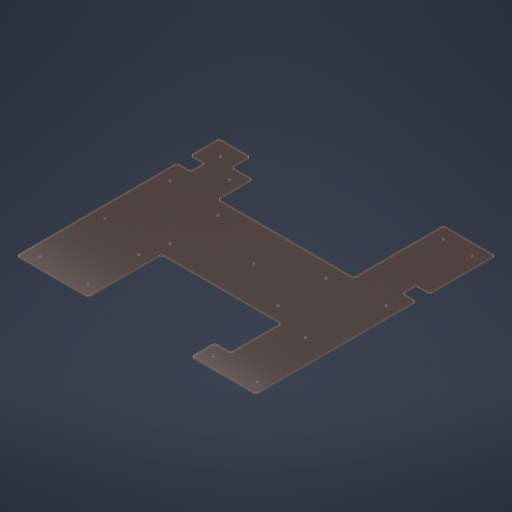
# Autodesk Inventor part: DB1-023
Saved by Autodesk Inventor 2023.4 (Build 274418000, 418)
## iProperties
Created: 2025-03-10
Part Number: DB1-023
Material: Polycarbonate, Smoke
Document SubType Name: Sheet Metal
Designer: brand
Density: 1.2 g/cm^3
Sheet Metal Rule: Default
Appearance: Polycarbonate - Smoked
Author: brand
Autodesk Inventor part; units mm, degrees
ref_plane "YZ Plane" through (0, 0, 0) normal (1, 0, 0) x (0, 1, 0)
ref_plane "XZ Plane" through (0, 0, 0) normal (0, 1, 0) x (-1, 0, 0)
ref_plane "XY Plane" through (0, 0, 0) normal (0, 0, 1) x (1, 0, 0)
sketch "Sketch1" plane through (0, 0, 0) normal (0, 1, 0) x (-1, 0, 0)
  line L0 (329.819, 329.819) -> (-329.819, 329.819)
  line L1 (-329.819, 329.819) -> (-329.819, -329.819)
  line L2 (-329.819, -329.819) -> (329.819, -329.819)
  line L3 (329.819, -329.819) -> (329.819, 329.819)
  line L4 (329.819, 329.819) -> (-329.819, -329.819) construction
  line L5 (-329.819, 329.819) -> (329.819, -329.819) construction
  line L6 (133.35, 329.819) -> (-133.35, 329.819) construction
  line L7 (-133.35, 329.819) -> (-133.35, 126.619)
  line L8 (-133.35, 126.619) -> (133.35, 126.619)
  line L9 (133.35, 126.619) -> (133.35, 329.819)
  line L10 (187.325, -329.819) -> (-187.325, -329.819) construction
  line L11 (-187.325, -329.819) -> (-187.325, -82.169)
  line L12 (-187.325, -82.169) -> (187.325, -82.169)
  line L13 (187.325, -82.169) -> (187.325, -329.819)
  point P0 (0, 0)
  point P1 (0, 329.819)
  point P2 (0, 329.819)
  point P3 (0, -329.819)
  point P4 (0, -329.819)
  point P5 (-133.35, 329.819)
  dimension "d0" = 659.638
  dimension "d1" = 659.638
  dimension "d2" = 266.7
  dimension "d3" = 203.2
  dimension "d4" = 247.65
  dimension "d5" = 374.65
  constraints: 28 end point, 6 midpoint, 6 parallel, 3 horizontal, 3 perpendicular, 2 coincident, 2 point on line
  measures "d0" distance of L0.start L0.end
  measures "d1" distance of L2.end L0.start
  measures "d2" distance of L7.end L8.end
  measures "d3" distance of L8.end L6.start
  measures "d4" distance of L12.end L10.start
  measures "d5" distance of L11.end L12.end
extrude "Extrusion1" add sketch "Sketch1" along normal mid plane 3.175 contours L3 L2 L13 L12 L11 L1 L0 L7 L8 L9
sketch "Sketch2" plane through (0, 1.5875, 0) normal (0, 1, 0) x (1, 0, 0)
  circle A0 centre (-283.3124, 275.8316) radius 34.925 construction
  line L0 (329.819, 329.819) -> (329.819, -329.819) construction
  line L1 (329.819, -329.819) -> (133.35, -329.819) construction
  line L2 (133.35, -329.819) -> (133.35, -126.619) construction
  line L3 (133.35, -126.619) -> (-133.35, -126.619) construction
  line L4 (-133.35, -126.619) -> (-133.35, -329.819) construction
  line L5 (-133.35, -329.819) -> (-329.819, -329.819) construction
  line L6 (-329.819, -329.819) -> (-329.819, 329.819) construction
  line L7 (-329.819, 329.819) -> (-187.325, 329.819) construction
  line L8 (-187.325, 329.819) -> (-187.325, 82.169) construction
  line L9 (-187.325, 82.169) -> (187.325, 82.169) construction
  line L10 (187.325, 82.169) -> (187.325, 329.819) construction
  line L11 (187.325, 329.819) -> (329.819, 329.819) construction
  line L12 (-187.325, 329.819) -> (-329.819, 329.819) construction
  line L13 (-329.819, 329.819) -> (-187.325, 329.819)
  line L14 (-187.325, 329.819) -> (-187.325, 228.219)
  line L15 (-187.325, 228.219) -> (-329.819, 228.219)
  line L16 (-329.819, 228.219) -> (-329.819, 329.819)
  line L17 (329.819, -329.819) -> (133.35, -329.819) construction
  line L18 (133.35, -126.619) -> (152.4, -126.619)
  line L19 (152.4, -126.619) -> (152.4, -329.819)
  line L20 (152.4, -329.819) -> (133.35, -329.819)
  line L21 (133.35, -329.819) -> (133.35, -126.619)
  line L22 (-329.819, 329.819) -> (-329.819, -329.819) construction
  line L23 (-329.819, 149.606) -> (-291.719, 149.606)
  line L24 (-291.719, 149.606) -> (-291.719, 111.506)
  line L25 (-291.719, 111.506) -> (-329.819, 111.506)
  line L26 (-329.819, 111.506) -> (-329.819, 149.606)
  line L27 (329.819, 149.606) -> (291.719, 149.606)
  line L28 (291.719, 149.606) -> (291.719, 111.506)
  line L29 (291.719, 111.506) -> (329.819, 111.506)
  line L30 (329.819, 111.506) -> (329.819, 149.606)
  line L31 (152.4, -126.619) -> (196.85, -126.619)
  line L32 (196.85, -126.619) -> (196.85, -266.319)
  line L33 (196.85, -266.319) -> (152.4, -266.319)
  line L34 (152.4, -266.319) -> (152.4, -126.619)
  line L35 (-187.325, 82.169) -> (-187.325, 329.819) construction
  line L36 (-187.325, 228.219) -> (-244.475, 228.219)
  line L37 (-244.475, 228.219) -> (-244.475, 177.419)
  line L38 (-244.475, 177.419) -> (-187.325, 177.419)
  line L39 (-187.325, 177.419) -> (-187.325, 228.219)
  circle A1 centre (-219.075, 209.169) radius 19.05 construction
  point P0 (0, 0)
  point P1 (-329.819, 130.556)
  point P2 (152.4, -266.319)
  dimension "d9" = 69.85
  dimension "d10" = 46.5066
  dimension "d11" = 53.9874
  dimension "d12" = 101.6
  dimension "d16" = 19.05
  dimension "d17" = 460.375
  dimension "d18" = 38.1
  dimension "d19" = 38.1
  dimension "d20" = 63.5
  dimension "d21" = 63.5
  dimension "d28" = 38.1
  dimension "d29" = 31.75
  dimension "d30" = 120.65
  dimension "d31" = 57.15
  dimension "d32" = 50.8
  constraints: 48 end point, 13 parallel, 6 horizontal, 6 perpendicular, 4 point on line, 2 centre point, 2 horizontal alignment, 1 midpoint
  measures "d9" diameter of A0
  measures "d10" distance from line of L16 A0.centre
  measures "d11" distance from line of L7 A0.centre
  measures "d12" distance of L13.end L14.end
  measures "d16" distance of L2.end L18.end
  measures "d17" distance from line of L5 point (-329.819, 130.556)
  measures "d18" distance of L23.end L24.end
  measures "d19" distance of L24.end L25.end
  measures "d20" distance between parallel lines of L2 L32
  measures "d21" distance between parallel lines of L1 L33
  measures "d28" diameter of A1
  measures "d29" distance from line of L35 A1.centre
  measures "d30" distance from line of L7 A1.centre
  measures "d31" distance of L37.end L38.end
  measures "d32" distance of L36.end L37.end
extrude "Extrusion2" cut sketch "Sketch2" against normal through all
fillet "Fillet1" radius 5.715 24 edges at (-133.35, 0, 126.619) (329.819, 0, 329.819) (329.819, 0, -329.819) (187.325, 0, -329.819) (187.325, 0, -82.169) (-187.325, 0, -82.169) (-329.819, 0, 329.819) (-329.819, 0, -228.219) (152.4, 0, 329.819) (-329.819, 0, -149.606) (-291.719, 0, -149.606) (-291.719, 0, -111.506) (-329.819, 0, -111.506) (291.719, 0, -149.606) (291.719, 0, -111.506) (329.819, 0, -111.506) (329.819, 0, -149.606) (196.85, 0, 126.619) (196.85, 0, 266.319) (152.4, 0, 266.319) (-187.325, 0, -177.419) (-244.475, 0, -177.419) (-244.475, 0, -228.219) (-133.35, 0, 329.819)
sketch "Sketch4" plane through (0, 1.5875, 0) normal (0, 1, 0) x (1, 0, 0)
  arc A0 (324.104, -329.819) -> (329.819, -324.104) centre (324.104, -324.104) ccw construction
  line L0 (324.104, -329.819) -> (158.115, -329.819) construction
  arc A1 (152.4, -324.104) -> (158.115, -329.819) centre (158.115, -324.104) ccw construction
  line L1 (152.4, -324.104) -> (152.4, -272.034) construction
  arc A2 (158.115, -266.319) -> (152.4, -272.034) centre (158.115, -272.034) ccw construction
  line L2 (158.115, -266.319) -> (191.135, -266.319) construction
  arc A3 (191.135, -266.319) -> (196.85, -260.604) centre (191.135, -260.604) ccw construction
  line L3 (196.85, -260.604) -> (196.85, -132.334) construction
  arc A4 (196.85, -132.334) -> (191.135, -126.619) centre (191.135, -132.334) ccw construction
  line L4 (191.135, -126.619) -> (-127.635, -126.619) construction
  arc A5 (-127.635, -126.619) -> (-133.35, -132.334) centre (-127.635, -132.334) ccw construction
  line L5 (-133.35, -132.334) -> (-133.35, -324.104) construction
  arc A6 (-139.065, -329.819) -> (-133.35, -324.104) centre (-139.065, -324.104) ccw construction
  line L6 (-139.065, -329.819) -> (-324.104, -329.819) construction
  arc A7 (-329.819, -324.104) -> (-324.104, -329.819) centre (-324.104, -324.104) ccw construction
  line L7 (-329.819, -324.104) -> (-329.819, 105.791) construction
  arc A8 (-324.104, 111.506) -> (-329.819, 105.791) centre (-324.104, 105.791) ccw construction
  line L8 (-324.104, 111.506) -> (-297.434, 111.506) construction
  arc A9 (-297.434, 111.506) -> (-291.719, 117.221) centre (-297.434, 117.221) ccw construction
  line L9 (-291.719, 117.221) -> (-291.719, 143.891) construction
  arc A10 (-291.719, 143.891) -> (-297.434, 149.606) centre (-297.434, 143.891) ccw construction
  line L10 (-297.434, 149.606) -> (-324.104, 149.606) construction
  arc A11 (-329.819, 155.321) -> (-324.104, 149.606) centre (-324.104, 155.321) ccw construction
  line L11 (-329.819, 155.321) -> (-329.819, 222.504) construction
  arc A12 (-324.104, 228.219) -> (-329.819, 222.504) centre (-324.104, 222.504) ccw construction
  line L12 (-324.104, 228.219) -> (-250.19, 228.219) construction
  arc A13 (-244.475, 222.504) -> (-250.19, 228.219) centre (-250.19, 222.504) ccw construction
  line L13 (-244.475, 222.504) -> (-244.475, 183.134) construction
  arc A14 (-244.475, 183.134) -> (-238.76, 177.419) centre (-238.76, 183.134) ccw construction
  line L14 (-238.76, 177.419) -> (-193.04, 177.419) construction
  arc A15 (-187.325, 171.704) -> (-193.04, 177.419) centre (-193.04, 171.704) ccw construction
  line L15 (-187.325, 171.704) -> (-187.325, 87.884) construction
  arc A16 (-187.325, 87.884) -> (-181.61, 82.169) centre (-181.61, 87.884) ccw construction
  line L16 (-181.61, 82.169) -> (181.61, 82.169) construction
  arc A17 (181.61, 82.169) -> (187.325, 87.884) centre (181.61, 87.884) ccw construction
  line L17 (187.325, 87.884) -> (187.325, 324.104) construction
  arc A18 (193.04, 329.819) -> (187.325, 324.104) centre (193.04, 324.104) ccw construction
  line L18 (193.04, 329.819) -> (324.104, 329.819) construction
  arc A19 (329.819, 324.104) -> (324.104, 329.819) centre (324.104, 324.104) ccw construction
  line L19 (329.819, 324.104) -> (329.819, 155.321) construction
  arc A20 (324.104, 149.606) -> (329.819, 155.321) centre (324.104, 155.321) ccw construction
  line L20 (324.104, 149.606) -> (297.434, 149.606) construction
  arc A21 (297.434, 149.606) -> (291.719, 143.891) centre (297.434, 143.891) ccw construction
  line L21 (291.719, 143.891) -> (291.719, 117.221) construction
  arc A22 (291.719, 117.221) -> (297.434, 111.506) centre (297.434, 117.221) ccw construction
  line L22 (297.434, 111.506) -> (324.104, 111.506) construction
  arc A23 (329.819, 105.791) -> (324.104, 111.506) centre (324.104, 105.791) ccw construction
  line L23 (329.819, 105.791) -> (329.819, -324.104) construction
  line L24 (180.7845, -298.069) -> (301.4345, -298.069) construction
  line L25 (196.85, -260.604) -> (196.85, -132.334) construction
  line L26 (196.85, -196.469) -> (329.819, -196.469) construction
  line L27 (329.819, 105.791) -> (329.819, -324.104) construction
  line L28 (191.135, -126.619) -> (-127.635, -126.619) construction
  line L29 (31.75, -126.619) -> (0, 82.169) construction
  line L30 (-324.104, 155.321) -> (-250.19, 222.504) construction
  line L31 (-298.069, 60.706) -> (-298.069, -298.069) construction
  point P0 (0, 0)
  point P1 (149.225, 44.069)
  point P2 (149.225, -88.519)
  point P3 (-149.225, 44.069)
  point P4 (-149.225, -88.519)
  point P5 (15.875, -22.225)
  point P6 (298.069, 60.706)
  point P7 (298.069, 298.069)
  point P8 (219.075, 298.069)
  point P9 (-165.1, -158.369)
  point P10 (263.3345, -126.619)
  point P11 (-298.069, -118.6815)
  point P12 (-287.147, 188.9125)
  point P13 (152.4, -298.069)
  point P14 (241.1095, -298.069)
  point P15 (241.1095, -329.819)
  point P16 (263.3345, -196.469)
  point P17 (15.875, -22.225)
  point P18 (-165.1, -298.069)
  point P19 (-287.147, 188.9125)
  point P20 (-219.075, 145.669)
  point P21 (-215.9, 177.419)
  point P22 (-298.069, -118.6815)
  dimension "d33" = 120.65
  dimension "d34" = 31.75
  dimension "d35" = 31.75
  dimension "d36" = 31.75
  dimension "d37" = 31.75
  dimension "d38" = 31.75
  dimension "d39" = 50.8
  dimension "d40" = 38.1
  dimension "d41" = 38.1
  dimension "d42" = 38.1
  dimension "d43" = 38.1
  dimension "d44" = 31.75
  dimension "d45" = 31.75
  dimension "d46" = 31.75
  dimension "d47" = 31.75
  dimension "d48" = 31.75
  dimension "d49" = 31.75
  dimension "d50" = 50.8
  dimension "d51" = 31.75
  constraints: 11 midpoint, 10 end point, 7 vertical alignment, 5 horizontal alignment, 3 coincident, 2 horizontal, 1 point on line, 1 vertical
  measures "d33" distance of L24.end L24.start
  measures "d34" distance from line of L18 point (298.069, 298.069)
  measures "d35" distance from line of L19 point (298.069, 298.069)
  measures "d36" distance from line of L17 point (219.075, 298.069)
  measures "d37" distance from line of L18 point (219.075, 298.069)
  measures "d38" distance from line of L23 point (298.069, 60.706)
  measures "d39" distance from line of point (298.069, 60.706) L22
  measures "d40" distance from line of L17 point (149.225, 44.069)
  measures "d41" distance from line of L16 point (149.225, 44.069)
  measures "d42" distance from line of L4 point (149.225, -88.519)
  measures "d43" distance from line of L15 point (-149.225, 44.069)
  measures "d44" distance from line of L5 point (-165.1, -298.069)
  measures "d45" distance from line of L6 point (-165.1, -298.069)
  measures "d46" distance from line of L6 L31.end
  measures "d47" distance from line of L7 L31.end
  measures "d48" vertical distance of point (-219.075, 145.669) point (-215.9, 177.419)
  measures "d49" distance from line of L15 point (-219.075, 145.669)
  measures "d50" distance from line of L8 L31.start
  measures "d51" distance from line of L4 point (-165.1, -158.369)
hole "Hole1" at (-298.069, 1.5875, 298.069) at (301.4345, 1.5875, 298.069) at (149.225, 1.5875, -44.069) at (149.225, 1.5875, 88.519) at (-149.225, 1.5875, -44.069) at (-149.225, 1.5875, 88.519) at (15.875, 1.5875, 22.225) at (-298.069, 1.5875, -60.706) at (298.069, 1.5875, -60.706) at (298.069, 1.5875, -298.069) at (219.075, 1.5875, -298.069) at (-165.1, 1.5875, 158.369) at (180.7845, 1.5875, 298.069) at (263.3345, 1.5875, 126.619) at (-298.069, 1.5875, 118.6815) at (-287.147, 1.5875, -188.9125) at (-165.1, 1.5875, 298.069) at (-219.075, 1.5875, -145.669) direction (0, -1, 0) diameter 5.1054 end through all clearance for "Flat Head Machine Screw (82)" size "#10" standard "Ansi Unified Screw Threads"
equation "\"d19\" = d18"
equation "\"d35\" = d34"
equation "\"d36\" = d34"
equation "\"d37\" = d34"
equation "\"d38\" = d36"
equation "\"d42\" = d41"
equation "\"d43\" = d40"
equation "\"d44\" = d38"
equation "\"d45\" = d44"
equation "\"d46\" = d45"
equation "\"d47\" = d44"
equation "\"d49\" = d48"
equation "\"d57\" = Thickness"
equation "\"BendRadius\" = Thickness"
equation "\"BendReliefWidth\" = Thickness"
equation "\"BendReliefDepth\" = 0.5 * Thickness"
equation "\"CornerReliefSize\" = 4 * Thickness"
equation "\"MinimumRemnant\" = 2 * Thickness"
equation "\"TransitionRadius\" = BendRadius"
equation "\"JacobiRadiusSize\" = BendRadius"
equation "\"GapSize\" = Thickness"
equation "\"Thickness\" = 3.048"
body "Solid1"
